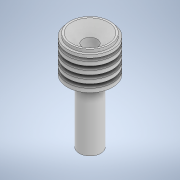
# Autodesk Inventor part: Barrel husillo 8mm_V2
Saved by Autodesk Inventor 2022 (Build 260153000, 153)
## iProperties
Created: 2022-02-10
Part Number: Barrel husillo 8mm_V2
Material: Genérico
Document SubType Name: Modeling
Designer: arman
Density: 1 g/cm^3
Appearance: Valor por defecto
Author: arman
Autodesk Inventor part; units mm, degrees
sketch "Boceto1" plane through (0, 0, 0) normal (0, 1, 0) x (-1, 0, 0)
  circle A0 centre (0, 0) radius 6
  circle A1 centre (0, 0) radius 3
  dimension "d0" = 12
  dimension "d1" = 6
  constraints: 2 centre point, 2 coincident
  measures "d0" diameter of A0
  measures "d1" diameter of A1
extrude "Extrusión1" add sketch "Boceto1" along normal blind 50
ref_plane "Plano de trabajo3" through (0, 7.5, 0) normal (0, 1, 0) x (1, 0, 0)
sketch "Boceto20" plane through (0, 50, 0) normal (0, 1, 0) x (1, 0, 0)
  circle A0 centre (0, 0) radius 7.75
  circle A1 centre (0, 0) radius 3.9641
  circle A2 centre (0, 0) radius 4
  dimension "d50" = 15.5
  dimension "d72" = 8
  constraints: 3 centre point, 3 coincident
  measures "d50" diameter of A0
  measures "d72" diameter of A2
extrude "Extrusión14" add sketch "Boceto20" along normal blind 1.6666 contours A0
sketch "Boceto21" plane through (0, 51.6666, 0) normal (0, 1, 0) x (1, 0, 0)
  circle A0 centre (0, 0) radius 12.5
  circle A1 centre (0, 0) radius 4
  dimension "d53" = 25
  constraints: 2 centre point, 2 coincident
  measures "d53" diameter of A0
extrude "Extrusión15" add sketch "Boceto21" along normal blind 1.6666
sketch "Boceto22" plane through (0, 53.3332, 0) normal (0, 1, 0) x (1, 0, 0)
  circle A0 centre (0, 0) radius 11.15
  circle A1 centre (0, 0) radius 3.9641
  dimension "d56" = 22.3
  constraints: 2 centre point, 2 coincident
  measures "d56" diameter of A0
extrude "Extrusión16" add sketch "Boceto22" along normal blind 1.6666
ref_plane "Plano de trabajo17" through (0, 43.5716, 0) normal (0, -1, 0) x (1, 0, 0)
ref_plane "Plano de trabajo16" through (0, 41.4287, 0) normal (0, -1, 0) x (1, 0, 0)
sketch "Boceto23" plane through (0, 35, 0) normal (0, -1, 0) x (1, 0, 0)
  circle A0 centre (0, 0) radius 12.5
  circle A1 centre (0, 0) radius 6
  dimension "d64" = 25
  dimension "d65" = 12
  constraints: 2 centre point, 2 coincident
  measures "d64" diameter of A0
  measures "d65" diameter of A1
extrude "Extrusión17" add sketch "Boceto23" against normal blind 2.1429
pattern_linear "Patrón rectangular1" count 4 spacing 4.2858 along (0, 1, 0) of "Extrusión17"
sketch "Boceto24" plane through (0, 54.9998, 0) normal (0, 1, 0) x (1, 0, 0)
  circle A0 centre (0, 0) radius 10.15
  dimension "d71" = 20.3
  constraints: 1 centre point, 1 coincident
  measures "d71" diameter of A0
ref_plane "Plano de trabajo18" through (0, 49.9998, 0) normal (0, 1, 0) x (1, 0, 0)
sketch "Boceto25" plane through (0, 49.9998, 0) normal (0, 1, 0) x (1, 0, 0)
  circle A0 centre (0, 0) radius 4
  dimension "d74" = 8
  constraints: 1 centre point, 1 coincident
  measures "d74" diameter of A0
loft "Solevación2" cut profiles "Boceto24", "Boceto25"
ref_plane "Plano de trabajo19" through (0, 7.5, 0) normal (0, -1, 0) x (1, 0, 0)
sketch "Boceto26" plane through (0, 7.5, 0) normal (0, -1, 0) x (1, 0, 0)
  circle A0 centre (0, 0) radius 6 projected
  circle A1 centre (0, 0) radius 4
  dimension "d80" = 8
  constraints: 1 centre point, 1 coincident
  measures "d80" diameter of A1
extrude "Extrusión18" cut sketch "Boceto26" against normal blind 47.5 contours A1
ref_plane "Plano de trabajo13" through (0, 35, 0) normal (0, -1, 0) x (1, 0, 0)
ref_plane "Plano de trabajo14" through (0, 37.1429, 0) normal (0, -1, 0) x (1, 0, 0)
ref_plane "Plano de trabajo15" through (0, 39.2858, 0) normal (0, -1, 0) x (1, 0, 0)
